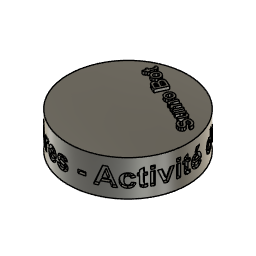
Socle v3 (Autodesk Fusion 360 design; units mm, degrees)
Autodesk Fusion 360 part; units mm, degrees
sketch "Esquisse1" plane through (0, 0, 0) normal (0, 0, 1) x (1, 0, 0)
  circle A0 centre (0, 0) radius 20
  dimension "d1" = 40
  constraint coincident A0.centre origin
  measures "d1" diameter of A0
extrude "Extrusion1" add sketch "Esquisse1" along normal blind 12
ref_plane "Plan de construction1" through (0, -20, 0) normal (0, 1, 0) x (0, 0, 1)
sketch "Esquisse2" plane through (0, -20, 0) normal (0, 1, 0) x (1, 0, 0)
  line L0 (-74.871, 8.8222) -> (161.6054, 8.8222) construction
  line L1 (161.6054, 8.8222) -> (161.6054, -21.1778) construction
  line L2 (161.6054, -21.1778) -> (-74.871, -21.1778) construction
  line L3 (-74.871, -21.1778) -> (-74.871, 8.8222) construction
  dimension "d5" = 5.9
  text T0 "Ares - Activité de rentrée 2021 -" font "Arial" height 5.9 bold align centre middle in box 236.4764 x 30 at (-74.871, 8.8222) x (1, 0) y (0, -1) spacing 1 kerned
emboss "Gravure en relief1" depth -1 profiles "Esquisse2" section 1 text T0 onto face at (19.9751, -0.9969, 8)
ref_plane "Plan de construction2" through (0, 0, 12) normal (0, 0, 1) x (1, 0, 0)
sketch "Esquisse3" plane through (0, 0, 12) normal (0, 0, 1) x (1, 0, 0)
  line L0 (20.0971, 8.1099) -> (-6.845, 20.3746) construction
  line L1 (-6.845, 20.3746) -> (-11.5013, 10.1458) construction
  line L2 (-11.5013, 10.1458) -> (15.4407, -2.1188) construction
  line L3 (15.4407, -2.1188) -> (20.0971, 8.1099) construction
  dimension "d11" = 4
  text T0 "Sumo Bot" font "Arial" height 4 bold align centre middle in box 29.6023 x 11.2387 at (20.0971, 8.1099) x (-0.910135, 0.414313) y (-0.414313, -0.910135) spacing 1 kerned
emboss "Gravure en relief2" depth 1 profiles "Esquisse3" section 1 text T0 onto face at (4.7423, -7.1112, 12)
